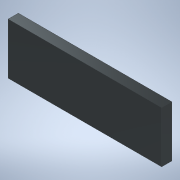
# Autodesk Inventor part: B_centro
Saved by Autodesk Inventor 2020 (Build 240168000, 168)
## iProperties
Created: 2020-07-18
Part Number: B_centro
Material: Hierro, fundido
Document SubType Name: Modeling
Designer: louis
Density: 7.15 g/cm^3
Appearance: Gris hierro
Author: louis
Autodesk Inventor part; units mm, degrees
ref_plane "YZ Plane" through (0, 0, 0) normal (1, 0, 0) x (0, 1, 0)
ref_plane "XZ Plane" through (0, 0, 0) normal (0, 1, 0) x (-1, 0, 0)
ref_plane "XY Plane" through (0, 0, 0) normal (0, 0, 1) x (1, 0, 0)
sketch "Boceto1" plane through (0, 0, 0) normal (0, 0, 1) x (1, 0, 0)
  line L0 (-64.7447, -49.4048) -> (85.2553, -49.4048)
  line L1 (85.2553, -49.4048) -> (85.2553, -99.4048)
  line L2 (85.2553, -99.4048) -> (-64.7447, -99.4048)
  line L3 (-64.7447, -99.4048) -> (-64.7447, -49.4048)
  point P0 (0, 0)
  point P1 (-14.8048, 10)
  dimension "d0" = 150
  dimension "d1" = 50
  constraints: 8 end point, 2 parallel, 1 horizontal, 1 perpendicular
  measures "d0" distance of L0.start L0.end
  measures "d1" distance of L2.end L0.start
extrude "Extrusión1" add sketch "Boceto1" along normal blind 10
